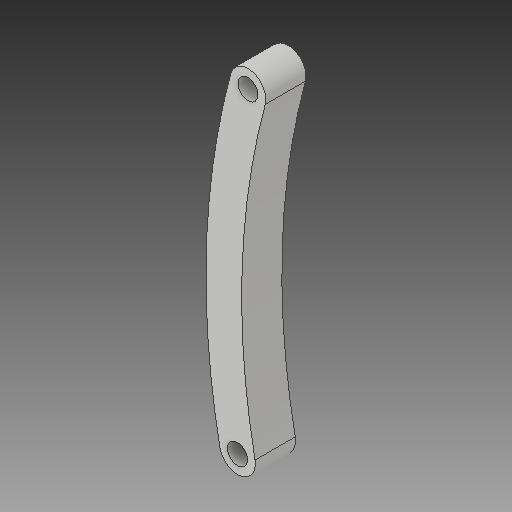
# Autodesk Inventor part: MasiveBone2
Saved by Autodesk Inventor 2017 (Build 210142000, 142)
## iProperties
Created: 2020-09-06
Part Number: MasiveBone2
Material: Generic
Document SubType Name: Modeling
Designer: agustin
Density: 1 g/cm^3
Appearance: Default
Author: agustin
Autodesk Inventor part; units mm, degrees
ref_plane "YZ Plane" through (0, 0, 0) normal (1, 0, 0) x (0, 1, 0)
ref_plane "XZ Plane" through (0, 0, 0) normal (0, 1, 0) x (-1, 0, 0)
ref_plane "XY Plane" through (0, 0, 0) normal (0, 0, 1) x (1, 0, 0)
sketch "Sketch1" plane through (0, 0, 0) normal (0, 0, 1) x (1, 0, 0)
  circle A0 centre (-23.5281, 14.2673) radius 2.25 projected
  circle A1 centre (-21.1834, 86.2291) radius 2.25 projected
  arc A2 (-21.1834, 86.2291) -> (-23.5281, 14.2673) centre (131.108, 45.2479) ccw construction
  arc A3 (-25.046, 87.2685) -> (-27.4502, 13.4815) centre (131.108, 45.2479) ccw
  arc A4 (-17.3208, 85.1897) -> (-19.6061, 15.053) centre (131.108, 45.2479) ccw
  arc A5 (-17.3208, 85.1897) -> (-25.046, 87.2685) centre (-21.1834, 86.2291) ccw
  arc A6 (-27.4502, 13.4815) -> (-19.6061, 15.053) centre (-23.5281, 14.2673) ccw
  point P0 (0, 0)
  dimension "d0" = 8
  constraints: 10 point on circle, 5 centre point, 4 tangent
  measures "d0" diameter of A5
extrude "Extrusion1" add sketch "Sketch1" along normal blind 9
scale "Scale1" factors (0.5, 0.5, 0.5) then translate (65.554, 22.624, 2.25) bodies 1
body "Solid1"
